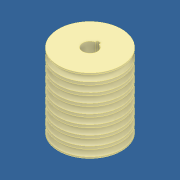
# Autodesk Inventor part: Roller
Saved by Autodesk Inventor 2018 (Build 220112000, 112)
## iProperties
Created: 2022-02-22
Part Number: Roller
Material: Nylon 6/6
Document SubType Name: Modeling
Designer: Nathann
Density: 1.13 g/cm^3
Appearance: Nylon 6
Mass: 34.2116 g
Surface Area: 84.9278 cm^2
Volume: 30.2757 cm^3
Author: Nathann
Autodesk Inventor part; units mm, degrees
ref_plane "YZ Plane" through (0, 0, 0) normal (1, 0, 0) x (0, 1, 0)
ref_plane "XZ Plane" through (0, 0, 0) normal (0, 1, 0) x (-1, 0, 0)
ref_plane "XY Plane" through (0, 0, 0) normal (0, 0, 1) x (1, 0, 0)
sketch "Sketch1" plane through (0, 0, 0) normal (0, 0, 1) x (1, 0, 0)
  circle A0 centre (0, 0) radius 17
  circle A1 centre (0, 0) radius 4
  dimension "d0" = 8
  dimension "d1" = 34
  constraints: 2 centre point, 2 coincident
  measures "d0" diameter of A1
  measures "d1" diameter of A0
extrude "Extrusion1" add sketch "Sketch1" along normal mid plane 40
sketch "Sketch2" plane through (0, 0, 20) normal (0, 0, 1) x (1, 0, 0)
  line L0 (0, 0) -> (5.2188, 0)
  line L1 (1, 3.8313) -> (-1, 3.8313)
  line L2 (-1, 3.8313) -> (-1, 5)
  line L3 (-1, 5) -> (1, 5)
  line L4 (1, 5) -> (1, 3.8313)
  line L5 (-1, 4) -> (1, 4)
  dimension "d31" = 2
  dimension "d32" = 1
  dimension "d33" = 4
  dimension "d34" = 1
  constraints: 12 end point, 3 horizontal, 2 parallel, 2 point on line, 1 perpendicular
  measures "d31" distance of L1.start L1.end
  measures "d32" horizontal distance of L0.start L1.start
  measures "d33" distance from line of L0.start L5
  measures "d34" distance between parallel lines of L3 L5
extrude "Extrusion2" cut sketch "Sketch2" against normal through all
sketch "Sketch3" plane through (0, 0, 20) normal (0, 0, 1) x (1, 0, 0)
  line L0 (-15.216, 3.5) -> (-15.216, -3.5)
  line L1 (-15.216, -3.5) -> (-7.216, 0)
  line L2 (-7.216, 0) -> (-15.216, 3.5)
  line L3 (-14.9274, -4.5769) -> (-11.4274, -10.6391)
  line L4 (-11.4274, -10.6391) -> (-6.2492, -3.608)
  line L5 (-6.2492, -3.608) -> (-14.9274, -4.5769)
  line L6 (-10.6391, -11.4274) -> (-4.5769, -14.9274)
  line L7 (-4.5769, -14.9274) -> (-3.608, -6.2492)
  line L8 (-3.608, -6.2492) -> (-10.6391, -11.4274)
  line L9 (-3.5, -15.216) -> (3.5, -15.216)
  line L10 (3.5, -15.216) -> (0, -7.216)
  line L11 (0, -7.216) -> (-3.5, -15.216)
  line L12 (4.5769, -14.9274) -> (10.6391, -11.4274)
  line L13 (10.6391, -11.4274) -> (3.608, -6.2492)
  line L14 (3.608, -6.2492) -> (4.5769, -14.9274)
  line L15 (11.4274, -10.6391) -> (14.9274, -4.5769)
  line L16 (14.9274, -4.5769) -> (6.2492, -3.608)
  line L17 (6.2492, -3.608) -> (11.4274, -10.6391)
  line L18 (15.216, -3.5) -> (15.216, 3.5)
  line L19 (15.216, 3.5) -> (7.216, 0)
  line L20 (7.216, 0) -> (15.216, -3.5)
  line L21 (14.9274, 4.5769) -> (11.4274, 10.6391)
  line L22 (11.4274, 10.6391) -> (6.2492, 3.608)
  line L23 (6.2492, 3.608) -> (14.9274, 4.5769)
  line L24 (10.6391, 11.4274) -> (4.5769, 14.9274)
  line L25 (4.5769, 14.9274) -> (3.608, 6.2492)
  line L26 (3.608, 6.2492) -> (10.6391, 11.4274)
  line L27 (3.5, 15.216) -> (-3.5, 15.216)
  line L28 (-3.5, 15.216) -> (0, 7.216)
  line L29 (0, 7.216) -> (3.5, 15.216)
  line L30 (-4.5769, 14.9274) -> (-10.6391, 11.4274)
  line L31 (-10.6391, 11.4274) -> (-3.608, 6.2492)
  line L32 (-3.608, 6.2492) -> (-4.5769, 14.9274)
  line L33 (-11.4274, 10.6391) -> (-14.9274, 4.5769)
  line L34 (-14.9274, 4.5769) -> (-6.2492, 3.608)
  line L35 (-6.2492, 3.608) -> (-11.4274, 10.6391)
  point P0 (0, 0)
  dimension "d9" = 7
  dimension "d10" = 8
  dimension "d11" = 3.5
  dimension "d14" = 360
  constraints: 72 end point, 1 vertical, 73 other
  measures "d9" distance of L0.start L0.end
  measures "d10" distance from line of L1.end L0
  measures "d11" vertical distance of L0.end point (0, 0)
extrude "Extrusion3" [suppressed]
sketch "Sketch4" plane through (0, 0, 0) normal (1, 0, 0) x (0, 1, 0)
  line L0 (-17, -20) -> (-17, 20) projected
  circle A0 centre (-17, -17.5) radius 1.75
  line L1 (-17, -20) -> (17, -20) projected
  line L2 (-17, -20) -> (-17, -23.2548)
  circle A1 centre (-17, -12.5) radius 1.75
  circle A2 centre (-17, -7.5) radius 1.75
  circle A3 centre (-17, -2.5) radius 1.75
  circle A4 centre (-17, 2.5) radius 1.75
  circle A5 centre (-17, 7.5) radius 1.75
  circle A6 centre (-17, 12.5) radius 1.75
  line L3 (17, -20) -> (17, -14.1403)
  line L4 (0, -32.2058) -> (0, 30.451) projected
  circle A7 centre (-17, 17.5) radius 1.75
  point P0 (0, 0)
  dimension "d18" = 2.5
  dimension "d19" = 3.5
  dimension "d22" = 5
  dimension "d27" = 34
  constraints: 8 centre point, 4 end point, 3 vertical, 1 point on line, 14 other
  measures "d18" distance from line of A0.centre L1
  measures "d19" diameter of A0
  measures "d22" distance of A0.centre A1.centre
  measures "d27" distance between parallel lines of L3 L2
revolve "Revolution1" cut sketch "Sketch4" angle 360 about axis through (0, 0, -10) along (0, 0, 1)
equation "\"d32\" = 0.5 * d31"
equation "\"d11\" = 0.5 * d9"
body "Solid1"
